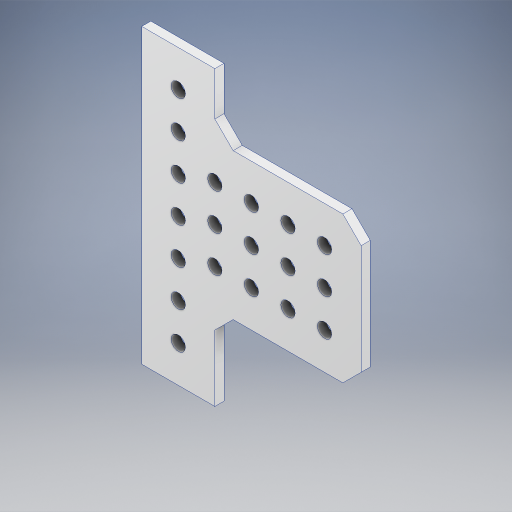
# Autodesk Inventor part: Custom-Underside-L-Gusset
Saved by Autodesk Inventor 2024.2 (Build 282272000, 272)
## iProperties
Created: 2024-02-11
Part Number: Custom-Underside-L-Gusset
Material: Aluminum 6061
Document SubType Name: Modeling
Designer: rohan
Density: 2.7 g/cm^3
Appearance: Aluminum - Flat
Author: rohan
Autodesk Inventor part; units mm, degrees
ref_plane "YZ Plane" through (0, 0, 0) normal (1, 0, 0) x (0, 1, 0)
ref_plane "XZ Plane" through (0, 0, 0) normal (0, 1, 0) x (-1, 0, 0)
ref_plane "XY Plane" through (0, 0, 0) normal (0, 0, 1) x (1, 0, 0)
sketch "Sketch1" plane through (0, 0, 0) normal (0, 0, 1) x (1, 0, 0)
  circle A0 centre (0, 0) radius 2.4892
  circle A1 centre (-12.7, 8.7884) radius 2.4892
  line L0 (-20.7225, -6.5967) -> (-20.7225, -16.769) construction
  line L1 (-24.8179, -11.6828) -> (-17.0895, -11.6828) construction
  circle A2 centre (-12.7, 21.4884) radius 2.4892
  circle A3 centre (-12.7, 34.1884) radius 2.4892
  circle A4 centre (-12.7, 46.8884) radius 2.4892
  circle A5 centre (12.7, 0) radius 2.4892
  circle A6 centre (25.4, 0) radius 2.4892
  circle A7 centre (38.1, 0) radius 2.4892
  circle A8 centre (0, -12.7) radius 2.4892
  circle A9 centre (12.7, -12.7) radius 2.4892
  circle A10 centre (25.4, -12.7) radius 2.4892
  circle A11 centre (38.1, -12.7) radius 2.4892
  circle A12 centre (-12.7, -3.9116) radius 2.4892
  circle A13 centre (0, -25.4) radius 2.4892
  circle A14 centre (12.7, -25.4) radius 2.4892
  circle A15 centre (25.4, -25.4) radius 2.4892
  circle A16 centre (38.1, -25.4) radius 2.4892
  circle A17 centre (-12.7, -16.6116) radius 2.4892
  circle A18 centre (-12.7, -29.3116) radius 2.4892
  circle A19 centre (-12.7, -42.0116) radius 2.4892
  line L2 (38.1, 0) -> (38.1, 12.7)
  line L3 (38.1, 12.7) -> (44.45, 12.7)
  line L4 (50.8, 12.7) -> (6.35, 12.7)
  line L5 (6.35, -38.1) -> (44.45, -38.1)
  line L6 (50.8, -31.75) -> (50.8, 6.35)
  line L7 (0, -44.45) -> (0, -54.7116)
  line L8 (-25.4, -54.7116) -> (-25.4, 34.1884)
  line L9 (0, 34.1884) -> (0, 19.05)
  line L10 (0, 19.05) -> (6.35, 12.7)
  line L11 (6.35, -38.1) -> (0, -44.45)
  line L12 (44.45, -38.1) -> (50.8, -31.75)
  line L13 (44.45, 12.7) -> (50.8, 6.35)
  circle A20 centre (-12.7, -54.7116) radius 2.4892
  line L14 (-12.7, 21.4884) -> (-12.7, 34.1884)
  line L15 (-12.7, 34.1884) -> (-25.4, 34.1884)
  line L16 (-25.4, 34.1884) -> (-25.4, 34.1884)
  line L17 (-12.7, 34.1884) -> (0, 34.1884)
  line L18 (0, 34.1884) -> (0, 34.1884)
  line L19 (0, -49.5808) -> (0, -67.4116)
  line L20 (0, -67.4116) -> (-25.4, -67.4116)
  line L21 (-25.4, -67.4116) -> (-25.4, -54.7116)
  point P0 (0, -38.1)
  point P1 (0, 12.7)
  point P2 (50.8, -38.1)
  dimension "d0" = 4.9784
  dimension "d1" = 4.9784
  dimension "d2" = 8.7884
  dimension "d3" = 12.7
  dimension "d6" = 12.7
  dimension "d13" = 12.7
  dimension "d28" = 12.7
  dimension "d35" = 12.7
  dimension "d42" = 12.7
  dimension "d43" = 12.7
  dimension "d44" = 50.8
  dimension "d45" = 16.6116
  dimension "d46" = 25.4
  dimension "d47" = 88.9
  dimension "d48" = 6.35
  dimension "d49" = 6.35
  dimension "d50" = 6.35
  dimension "d51" = 6.35
  dimension "d52" = 6.35
  dimension "d53" = 6.35
  dimension "d54" = 6.35
  dimension "d55" = 6.35
  dimension "d60" = 12.7
  dimension "d66" = 12.7
  constraints: 44 end point, 21 centre point, 12 point on line, 8 vertical, 6 perpendicular, 3 horizontal, 1 coincident, 1 midpoint, 1 parallel, 38 other
  measures "d0" diameter of A0
  measures "d1" diameter of A1
  measures "d2" vertical distance of A1.centre point (0, 0)
  measures "d3" horizontal distance of A1.centre point (0, 0)
  measures "d6" distance of A1.centre L14.start
  measures "d13" distance of A0.centre A5.centre
  measures "d28" distance of A0.centre A8.centre
  measures "d35" distance of A17.centre A18.centre
  measures "d42" distance of L2.start L2.end
  measures "d43" distance of L2.end L4.start
  measures "d44" distance of point (0, -38.1) point (0, 12.7)
  measures "d45" distance of point (0, -38.1) L7.end
  measures "d46" distance of L7.end L8.start
  measures "d47" distance of L8.start L8.end
  measures "d48" distance of L9.end point (0, 12.7)
  measures "d49" distance of L4.end point (0, 12.7)
  measures "d50" distance of L5.start point (0, -38.1)
  measures "d51" distance of L7.start point (0, -38.1)
  measures "d52" distance of L5.end point (50.8, -38.1)
  measures "d53" distance of L6.start point (50.8, -38.1)
  measures "d54" distance of L3.end L4.start
  measures "d55" distance of L6.end L4.start
  measures "d60" distance of A19.centre A20.centre
  measures "d66" distance from line of L20 A20.centre
extrude "Extrusion2" add sketch "Sketch1" along normal blind 3.175 contours L17 L9 L10 L4 L3 L13 L6 L12 L5 L11 L7 L19 L20 L21 L8 L15 A3 | A3 L14 L17 | L15 L14 A3
equation "\"d49\" = d48"
equation "\"d51\" = d50"
equation "\"d53\" = d52"
equation "\"d54\" = d52"
equation "\"d55\" = d54"
body "Solid2"
